Leg v6 (Autodesk Fusion 360 design; units mm, degrees)
Autodesk Fusion 360 part; units mm, degrees
sketch "RobotSatan_Outline_2" plane through (0, 0, 0) normal (0, 1, 0) x (1, 0, 0)
  spline S0 degree 3 poles (-4.0018, -2.6368) (-4.0018, -2.6368) (-1.7304, -4.4815) (0.4503, -4.3985) knots 0 0 0 0 1 1 1 1 construction
  spline S1 degree 3 poles (63.629, -4.044) (65.7695, -3.9442) (67.8342, -1.9163) (67.8342, -1.9163) knots 0 0 0 0 1 1 1 1 construction
  spline S2 degree 3 poles (61.8838, 8.3153) (62.2969, 9.5277) (62.4552, 13.6834) (61.5349, 14.1566) knots 0 0 0 0 1 1 1 1 construction
  spline S3 degree 3 poles (67.8342, -1.9163) (67.8342, -1.9163) (70.4644, 0.8212) (71.1371, 2.4758) knots 0 0 0 0 1 1 1 1 construction
  spline S4 degree 3 poles (4.7919, 41.52) (1.6976, 37.0721) (-0.1427, 30.975) (-0.3241, 24.5701) knots 0 0 0 0 1 1 1 1 construction
  spline S5 degree 3 poles (-7.7347, 1.4577) (-6.9084, -0.1335) (-4.0018, -2.6368) (-4.0018, -2.6368) knots 0 0 0 0 1 1 1 1 construction
  spline S6 degree 3 poles (25.4469, 4.8587) (26.757, 5.8451) (29.0105, 9.0389) (28.1329, 10.0991) knots 0 0 0 0 1 1 1 1 construction
  spline S7 degree 3 poles (0.9949, 13.9146) (0.1024, 13.3642) (0.6239, 9.2378) (1.1482, 8.0651) knots 0 0 0 0 1 1 1 1 construction
  line L0 (61.8838, 8.3153) -> (69.5308, 5.8795) construction
  spline S8 degree 3 poles (16.1754, 48.2878) (11.9809, 48.4024) (7.8861, 45.9679) (4.7919, 41.52) knots 0 0 0 0 1 1 1 1 construction
  spline S9 degree 3 poles (61.5349, 14.1566) (62.1985, 17.5571) (62.3292, 21.2262) (61.9169, 24.8838) knots 0 0 0 0 1 1 1 1 construction
  spline S10 degree 3 poles (-6.4002, 4.9865) (-6.4002, 4.9865) (-8.5609, 3.0488) (-7.7347, 1.4577) knots 0 0 0 0 1 1 1 1 construction
  spline S11 degree 3 poles (0.4503, -4.3985) (2.6311, -4.3154) (22.3185, -1.4309) (23.4492, 0.0355) knots 0 0 0 0 1 1 1 1 construction
  spline S12 degree 3 poles (43.7533, 47.1341) (37.1756, 46.3732) (32.0634, 39.2113) (31.0191, 29.2946) knots 0 0 0 0 1 1 1 1 construction
  line L1 (1.1482, 8.0651) -> (-6.4002, 4.9865) construction
  spline S13 degree 3 poles (71.1371, 2.4758) (71.8098, 4.1303) (69.5308, 5.8795) (69.5308, 5.8795) knots 0 0 0 0 1 1 1 1 construction
  spline S14 degree 3 poles (38.385, 3.0871) (38.9879, 1.5836) (39.975, -0.6905) (40.7508, -1.5514) knots 0 0 0 0 1 1 1 1 construction
  spline S15 degree 3 poles (40.7508, -1.5514) (41.982, -2.9178) (61.4884, -4.1438) (63.629, -4.044) knots 0 0 0 0 1 1 1 1 construction
  spline S16 degree 3 poles (-0.3241, 24.5701) (-0.4249, 20.8907) (0.0263, 17.2461) (0.9949, 13.9146) knots 0 0 0 0 1 1 1 1 construction
  spline S17 degree 3 poles (23.4492, 0.0355) (24.1617, 0.9594) (24.9655, 3.3093) (25.4469, 4.8587) knots 0 0 0 0 1 1 1 1 construction
  spline S18 degree 3 poles (31.1122, 20.9238) (31.7006, 16.2301) (33.1605, 11.7653) (35.3109, 8.0833) knots 0 0 0 0 1 1 1 1 construction
  spline S19 degree 3 poles (31.0191, 29.2946) (29.6368, 40.2178) (23.4961, 48.0751) (16.1754, 48.2878) knots 0 0 0 0 1 1 1 1 construction
  spline S20 degree 3 poles (28.1329, 10.0991) (29.6834, 13.3051) (30.7062, 17.0213) (31.1122, 20.9238) knots 0 0 0 0 1 1 1 1 construction
  spline S21 degree 3 poles (61.9169, 24.8838) (60.4852, 37.482) (53.0344, 47.225) (44.8524, 47.1981) knots 0 0 0 0 1 1 1 1 construction
  spline S22 degree 3 poles (35.3109, 8.0833) (34.543, 6.9535) (37.0192, 3.9603) (38.385, 3.0871) knots 0 0 0 0 1 1 1 1 construction
  spline S23 degree 3 poles (44.8524, 47.1981) (44.4843, 47.1969) (44.1177, 47.1755) (43.7533, 47.1341) knots 0 0 0 0 1 1 1 1 construction
  spline S24 degree 5 poles (31.0191, 29.2946) (31.0111, 29.2894) (30.9933, 29.2931) (30.9604, 29.343) (30.9015, 29.5057) (30.7982, 29.8768) (30.6618, 30.4134) (30.4903, 31.1054) (30.2828, 31.9364) (30.0394, 32.8844) (29.7611, 33.9237) (29.4494, 35.0262) (29.1066, 36.1626) (28.7352, 37.3041) (28.338, 38.4234) (27.918, 39.4965) (27.4781, 40.5035) (27.0208, 41.431) (26.5487, 42.2711) (26.0639, 43.0212) (25.5684, 43.6827) (25.0637, 44.2606) (24.5515, 44.7626) (24.0328, 45.1982) (23.5086, 45.5782) (22.9796, 45.9134) (22.4464, 46.2145) (21.909, 46.4908) (21.3676, 46.7496) (20.8219, 46.9954) (20.2714, 47.2296) (19.7155, 47.4512) (19.1536, 47.6575) (18.585, 47.8443) (18.0094, 48.0066) (17.4263, 48.1391) (16.8357, 48.2366) (16.2379, 48.2949) (15.6336, 48.3107) (15.0238, 48.2827) (14.4104, 48.2111) (13.795, 48.0973) (13.1799, 47.9437) (12.5675, 47.7532) (11.96, 47.5293) (11.3598, 47.2753) (10.7691, 46.9943) (10.1899, 46.6888) (9.624, 46.3606) (9.0726, 46.0102) (8.5367, 45.6368) (8.017, 45.2393) (7.5137, 44.8154) (7.0269, 44.363) (6.5565, 43.8795) (6.102, 43.3625) (5.6629, 42.8101) (5.2387, 42.2208) (4.8287, 41.5939) (4.4321, 40.9297) (4.0482, 40.23) (3.6763, 39.4975) (3.3159, 38.7358) (2.9663, 37.9493) (2.6273, 37.1425) (2.2986, 36.3207) (1.9802, 35.4888) (1.6724, 34.6516) (1.3757, 33.8137) (1.0908, 32.9788) (0.8191, 32.1501) (0.562, 31.3295) (0.3215, 30.5177) (0.1, 29.7142) (-0.0996, 28.9165) (-0.2743, 28.1212) (-0.4207, 27.3241) (-0.536, 26.5206) (-0.6172, 25.7065) (-0.6623, 24.8778) (-0.6696, 24.0319) (-0.6387, 23.1674) (-0.5701, 22.2848) (-0.4654, 21.387) (-0.3281, 20.4794) (-0.1632, 19.571) (0.0225, 18.6739) (0.2201, 17.8048) (0.4185, 16.9835) (0.6063, 16.231) (0.7719, 15.5667) (0.9049, 15.0065) (0.9968, 14.5606) (1.042, 14.2311) (1.0388, 14.0095) (0.9901, 13.8752) (0.9047, 13.7922) (0.7973, 13.7097) (0.6851, 13.5785) (0.5842, 13.3649) (0.5088, 13.0503) (0.4701, 12.6295) (0.4753, 12.1101) (0.5262, 11.5114) (0.6185, 10.8629) (0.7407, 10.204) (0.876, 9.578) (1.0052, 9.0265) (1.1093, 8.5838) (1.1717, 8.2713) (1.1807, 8.0912) (1.1322, 8.0228) (1.0327, 8.0115) (0.8972, 7.9857) (0.7382, 7.921) (0.5625, 7.8283) (0.369, 7.728) (0.1458, 7.6264) (-0.1255, 7.5178) (-0.4648, 7.3903) (-0.8886, 7.2301) (-1.4057, 7.0265) (-2.0115, 6.7767) (-2.6848, 6.4899) (-3.3936, 6.1826) (-4.0992, 5.876) (-4.7615, 5.5924) (-5.3435, 5.352) (-5.8163, 5.1692) (-6.1636, 5.05) (-6.3871, 4.9878) (-6.5098, 4.9612) (-6.5847, 4.9281) (-6.6707, 4.8433) (-6.7961, 4.6861) (-6.9627, 4.4573) (-7.1567, 4.1701) (-7.3567, 3.8446) (-7.5443, 3.4995) (-7.7054, 3.15) (-7.8298, 2.8085) (-7.9105, 2.4837) (-7.9435, 2.1803) (-7.9276, 1.899) (-7.8635, 1.6359) (-7.754, 1.3841) (-7.6034, 1.1356) (-7.417, 0.8829) (-7.2008, 0.6209) (-6.9611, 0.3474) (-6.7041, 0.0626) (-6.4358, -0.2313) (-6.1612, -0.5311) (-5.8841, -0.8324) (-5.6068, -1.1306) (-5.33, -1.4212) (-5.0532, -1.7) (-4.776, -1.9634) (-4.4979, -2.2088) (-4.2193, -2.4347) (-3.9422, -2.6411) (-3.6705, -2.8298) (-3.4086, -3.0036) (-3.1594, -3.1658) (-2.9235, -3.3194) (-2.6971, -3.4672) (-2.4707, -3.6101) (-2.2323, -3.7483) (-1.9713, -3.8807) (-1.6808, -4.0054) (-1.3626, -4.1197) (-1.0273, -4.2204) (-0.6894, -4.3043) (-0.3635, -4.3684) (-0.06, -4.4107) (0.2192, -4.4301) (0.4846, -4.4277) (0.7549, -4.4053) (1.0522, -4.3659) (1.3972, -4.3126) (1.8047, -4.2485) (2.2802, -4.1762) (2.8216, -4.098) (3.4209, -4.0156) (4.0658, -3.9307) (4.7411, -3.8444) (5.4302, -3.7577) (6.1166, -3.6711) (6.7858, -3.5852) (7.4264, -3.5002) (8.0317, -3.4161) (8.6006, -3.3329) (9.1356, -3.2504) (9.6424, -3.1682) (10.1289, -3.0859) (10.6041, -3.0031) (11.0773, -2.9193) (11.557, -2.8339) (12.0504, -2.7463) (12.5617, -2.6561) (13.0932, -2.5628) (13.645, -2.4658) (14.2157, -2.365) (14.8026, -2.2599) (15.4022, -2.1504) (16.01, -2.0365) (16.6217, -1.9183) (17.2328, -1.7961) (17.8392, -1.6704) (18.4372, -1.5419) (19.0234, -1.4113) (19.5943, -1.2794) (20.1462, -1.1472) (20.6751, -1.0154) (21.1762, -0.8847) (21.6444, -0.7558) (22.0732, -0.629) (22.4551, -0.5047) (22.7823, -0.3827) (23.0491, -0.2627) (23.2538, -0.144) (23.4009, -0.0255) (23.5034, 0.0941) (23.5821, 0.2169) (23.6573, 0.3472) (23.7421, 0.4931) (23.8421, 0.6649) (23.9589, 0.8736) (24.0916, 1.1286) (24.238, 1.4367) (24.3945, 1.8003) (24.5567, 2.2164) (24.7193, 2.6747) (24.8766, 3.1566) (25.0229, 3.6331) (25.153, 4.0687) (25.2636, 4.4304) (25.3547, 4.6943) (25.431, 4.8544) (25.5023, 4.9287) (25.5865, 4.9705) (25.702, 5.0425) (25.8576, 5.1765) (26.0542, 5.3795) (26.2863, 5.643) (26.5442, 5.9509) (26.8158, 6.2885) (27.0881, 6.6445) (27.3482, 7.0094) (27.5846, 7.3755) (27.7883, 7.7361) (27.9542, 8.0852) (28.082, 8.4167) (28.1777, 8.7241) (28.2497, 9.0014) (28.3043, 9.2445) (28.3428, 9.452) (28.3543, 9.6267) (28.3198, 9.7759) (28.2352, 9.9073) (28.1424, 10.0247) (28.1125, 10.1292) (28.1686, 10.2278) (28.2589, 10.336) (28.3384, 10.4699) (28.4062, 10.6416) (28.4793, 10.8573) (28.5744, 11.1149) (28.6922, 11.4037) (28.8257, 11.7082) (28.9627, 12.0126) (29.0913, 12.3043) (29.2043, 12.5783) (29.3022, 12.8394) (29.3899, 13.0974) (29.4739, 13.3628) (29.5603, 13.6434) (29.6516, 13.939) (29.7464, 14.2424) (29.8414, 14.544) (29.9328, 14.8349) (30.0175, 15.1108) (30.0953, 15.3768) (30.1682, 15.6452) (30.2391, 15.9303) (30.3112, 16.2431) (30.386, 16.5867) (30.4628, 16.9503) (30.5386, 17.3134) (30.61, 17.654) (30.6737, 17.9546) (30.7279, 18.209) (30.7735, 18.4304) (30.8143, 18.6527) (30.8548, 18.9132) (30.8989, 19.2396) (30.948, 19.6357) (30.9989, 20.0659) (31.046, 20.471) (31.084, 20.7851) (31.1099, 20.9528) (31.125, 20.9445) (31.1381, 20.7771) (31.1614, 20.4992) (31.2015, 20.1593) (31.257, 19.7928) (31.3225, 19.425) (31.3901, 19.0714) (31.4534, 18.7382) (31.5088, 18.4237) (31.5597, 18.1183) (31.6142, 17.8079) (31.6818, 17.4778) (31.7711, 17.1163) (31.8868, 16.7185) (32.0268, 16.2903) (32.18, 15.8506) (32.3309, 15.4247) (32.4634, 15.0385) (32.5644, 14.7123) (32.6277, 14.455) (32.6576, 14.2585) (32.6737, 14.09) (32.7019, 13.9064) (32.7645, 13.671) (32.8676, 13.3723) (33.0016, 13.0247) (33.1492, 12.6556) (33.2908, 12.297) (33.4115, 11.9747) (33.5072, 11.6991) (33.5911, 11.4551) (33.6858, 11.2126) (33.8153, 10.9375) (33.9976, 10.6027) (34.2358, 10.1988) (34.5114, 9.7444) (34.7924, 9.2758) (35.0416, 8.8367) (35.2248, 8.4679) (35.3196, 8.1968) (35.3223, 8.0283) (35.2592, 7.9314) (35.186, 7.8396) (35.1473, 7.7015) (35.1511, 7.5126) (35.1875, 7.2909) (35.2458, 7.0538) (35.327, 6.8025) (35.4373, 6.5302) (35.5855, 6.2274) (35.779, 5.8874) (36.0193, 5.5123) (36.3012, 5.1148) (36.6145, 4.7134) (36.9452, 4.3294) (37.2769, 3.9837) (37.592, 3.6931) (37.8734, 3.4674) (38.1053, 3.3053) (38.2753, 3.193) (38.3802, 3.1082) (38.4305, 3.0249) (38.4579, 2.9172) (38.5006, 2.7655) (38.5761, 2.5645) (38.6835, 2.3206) (38.8123, 2.0468) (38.9486, 1.7575) (39.0838, 1.4639) (39.2143, 1.1727) (39.34, 0.8879) (39.4637, 0.6104) (39.5892, 0.3391) (39.7204, 0.0711) (39.8606, -0.1965) (40.0108, -0.4652) (40.1698, -0.7325) (40.3324, -0.9907) (40.4887, -1.2241) (40.6273, -1.4141) (40.741, -1.5488) (40.8312, -1.629) (40.9141, -1.679) (41.0117, -1.7285) (41.1388, -1.7875) (41.3038, -1.8535) (41.5087, -1.9227) (41.7511, -1.9933) (42.0259, -2.0637) (42.3276, -2.1336) (42.6519, -2.2027) (42.9967, -2.2709) (43.3612, -2.3383) (43.7457, -2.4051) (44.1511, -2.4716) (44.5782, -2.5378) (45.0279, -2.604) (45.5003, -2.6699) (45.9952, -2.7356) (46.5116, -2.8008) (47.0479, -2.8653) (47.602, -2.9287) (48.1709, -2.9909) (48.7506, -3.0514) (49.3364, -3.1101) (49.9228, -3.1667) (50.5038, -3.2211) (51.0735, -3.2731) (51.6264, -3.3227) (52.1582, -3.3698) (52.6659, -3.4144) (53.1483, -3.4565) (53.6066, -3.4962) (54.0446, -3.5336) (54.4691, -3.5688) (54.8881, -3.6021) (55.3097, -3.6335) (55.7415, -3.6634) (56.1886, -3.6921) (56.6534, -3.7199) (57.1335, -3.7472) (57.6219, -3.7745) (58.109, -3.8022) (58.5841, -3.8304) (59.0372, -3.8593) (59.4608, -3.8885) (59.8514, -3.9176) (60.2118, -3.9454) (60.5522, -3.9705) (60.887, -3.991) (61.2307, -4.0058) (61.594, -4.0141) (61.9799, -4.0166) (62.3794, -4.0153) (62.7692, -4.0144) (63.1214, -4.0177) (63.4113, -4.0275) (63.6264, -4.0427) (63.7743, -4.0574) (63.8925, -4.0584) (64.0263, -4.0338) (64.1962, -3.9855) (64.394, -3.927) (64.6018, -3.8725) (64.8064, -3.8247) (65.0063, -3.7731) (65.205, -3.7041) (65.4083, -3.6083) (65.6205, -3.4881) (65.8441, -3.3521) (66.0797, -3.2104) (66.3259, -3.0689) (66.5791, -2.9242) (66.834, -2.7677) (67.0841, -2.5905) (67.3228, -2.3881) (67.5437, -2.1655) (67.7412, -1.9413) (67.912, -1.7384) (68.0567, -1.5756) (68.1802, -1.46) (68.2946, -1.3756) (68.4141, -1.2927) (68.5485, -1.1848) (68.6977, -1.0404) (68.8564, -0.8598) (69.0166, -0.6528) (69.1722, -0.4364) (69.3198, -0.2295) (69.4587, -0.0462) (69.5911, 0.1099) (69.723, 0.2541) (69.8617, 0.413) (70.0127, 0.6105) (70.1758, 0.8543) (70.3431, 1.125) (70.5029, 1.3906) (70.6441, 1.619) (70.7595, 1.7903) (70.8514, 1.9138) (70.93, 2.0231) (71.0047, 2.1513) (71.0769, 2.3071) (71.142, 2.4806) (71.1947, 2.6563) (71.2328, 2.8234) (71.256, 2.978) (71.2649, 3.1263) (71.2596, 3.2836) (71.2402, 3.4608) (71.2062, 3.6458) (71.1575, 3.8109) (71.0967, 3.9366) (71.0318, 4.0377) (70.9712, 4.1506) (70.9096, 4.2933) (70.8309, 4.4574) (70.7255, 4.6233) (70.609, 4.771) (70.5069, 4.8902) (70.429, 4.987) (70.3414, 5.0957) (70.1989, 5.253) (69.9874, 5.4655) (69.7602, 5.6833) (69.5848, 5.8436) (69.5049, 5.9042) (69.4785, 5.8941) (69.377, 5.9175) (69.2074, 5.9796) (69.0289, 6.0454) (68.8687, 6.0968) (68.7112, 6.1417) (68.5308, 6.1943) (68.3148, 6.2617) (68.0659, 6.3427) (67.7933, 6.4325) (67.5087, 6.5252) (67.2182, 6.6179) (66.9232, 6.7108) (66.6226, 6.8053) (66.3152, 6.903) (66.0018, 7.0044) (65.6877, 7.107) (65.382, 7.2064) (65.0949, 7.2978) (64.8344, 7.3776) (64.6044, 7.4453) (64.401, 7.5052) (64.2136, 7.5653) (64.0269, 7.6331) (63.8224, 7.7128) (63.5816, 7.8026) (63.2922, 7.8974) (62.9553, 7.9908) (62.5906, 8.0774) (62.246, 8.1547) (61.9895, 8.2246) (61.8649, 8.2894) (61.8793, 8.3527) (61.9283, 8.4107) (61.9329, 8.4774) (61.9545, 8.5927) (61.995, 8.7507) (62.0358, 8.9242) (62.0638, 9.0923) (62.0829, 9.2506) (62.1005, 9.4028) (62.1198, 9.5578) (62.1391, 9.7238) (62.156, 9.9023) (62.1699, 10.0834) (62.1812, 10.2552) (62.1905, 10.4139) (62.1981, 10.5706) (62.2043, 10.7396) (62.209, 10.9281) (62.2118, 11.1312) (62.2124, 11.3395) (62.2103, 11.543) (62.205, 11.7356) (62.1964, 11.9151) (62.185, 12.0848) (62.1722, 12.2534) (62.1588, 12.4287) (62.1431, 12.6089) (62.1211, 12.7795) (62.0909, 12.9272) (62.0592, 13.0553) (62.0392, 13.1869) (62.0281, 13.342) (61.991, 13.5221) (61.894, 13.7146) (61.7371, 13.8994) (61.586, 14.0537) (61.5113, 14.1632) (61.5386, 14.2322) (61.5778, 14.2953) (61.5869, 14.3962) (61.6011, 14.5685) (61.6368, 14.8098) (61.6892, 15.0879) (61.7447, 15.3626) (61.7887, 15.6) (61.8174, 15.7946) (61.8365, 15.9635) (61.8543, 16.1294) (61.8757, 16.3032) (61.8996, 16.4804) (61.9233, 16.6553) (61.9453, 16.8339) (61.9665, 17.035) (61.9881, 17.2795) (62.0115, 17.5833) (62.0368, 17.9499) (62.0633, 18.3744) (62.0899, 18.8455) (62.115, 19.3479) (62.1367, 19.8655) (62.1532, 20.3834) (62.1631, 20.8908) (62.1649, 21.3832) (62.158, 21.8608) (62.1419, 22.3275) (62.1162, 22.7894) (62.0812, 23.2534) (62.0372, 23.726) (61.9849, 24.212) (61.9251, 24.7129) (61.859, 25.2265) (61.7875, 25.7479) (61.712, 26.2706) (61.6333, 26.7872) (61.5524, 27.2906) (61.4696, 27.7751) (61.3852, 28.2367) (61.2988, 28.675) (61.2092, 29.0932) (61.115, 29.4977) (61.0147, 29.8963) (60.9062, 30.298) (60.7877, 30.7111) (60.6575, 31.1431) (60.5142, 31.5991) (60.3566, 32.081) (60.1842, 32.5883) (59.9967, 33.1182) (59.794, 33.6667) (59.5765, 34.2283) (59.3449, 34.7973) (59.0998, 35.3676) (58.8426, 35.9335) (58.5743, 36.4903) (58.2966, 37.0343) (58.011, 37.5633) (57.719, 38.076) (57.4219, 38.5719) (57.1209, 39.0512) (56.8166, 39.515) (56.5094, 39.9643) (56.1987, 40.4008) (55.8836, 40.8262) (55.5622, 41.2421) (55.2317, 41.6502) (54.8893, 42.0517) (54.5317, 42.4476) (54.156, 42.8387) (53.7597, 43.2251) (53.3407, 43.6066) (52.8982, 43.9821) (52.4322, 44.3499) (51.9447, 44.7075) (51.4384, 45.0519) (50.9173, 45.3796) (50.3859, 45.687) (49.8489, 45.9705) (49.3114, 46.227) (48.7781, 46.4538) (48.2529, 46.6492) (47.7394, 46.8123) (47.2396, 46.9436) (46.7547, 47.0446) (46.2845, 47.1182) (45.828, 47.1671) (45.3838, 47.1945) (44.9496, 47.2033) (44.5229, 47.1955) (44.1009, 47.1722) (43.6811, 47.133) (43.2608, 47.0762) (42.8379, 46.9997) (42.4105, 46.9009) (41.9777, 46.7777) (41.5394, 46.6284) (41.0964, 46.4526) (40.651, 46.2514) (40.2062, 46.0273) (39.7658, 45.7836) (39.3338, 45.5239) (38.914, 45.2519) (38.5097, 44.9708) (38.1234, 44.683) (37.7562, 44.3893) (37.4076, 44.0891) (37.0759, 43.78) (36.7584, 43.4591) (36.4519, 43.123) (36.1533, 42.7686) (35.8596, 42.3938) (35.5689, 41.9975) (35.2804, 41.5808) (34.9945, 41.1466) (34.7128, 40.6994) (34.4376, 40.2445) (34.1715, 39.7873) (33.9172, 39.3332) (33.6772, 38.8863) (33.4533, 38.4496) (33.2466, 38.024) (33.0569, 37.6077) (32.883, 37.1974) (32.7233, 36.7885) (32.5756, 36.3763) (32.4375, 35.9568) (32.3067, 35.527) (32.1813, 35.086) (32.0601, 34.6359) (31.9421, 34.1808) (31.8273, 33.7266) (31.716, 33.2791) (31.6089, 32.8438) (31.5074, 32.4249) (31.4131, 32.024) (31.3279, 31.6394) (31.2541, 31.2664) (31.1934, 30.9005) (31.1467, 30.5399) (31.1132, 30.1881) (31.0904, 29.8569) (31.0731, 29.5691) (31.0576, 29.4003) (31.0412, 29.3241) (31.0271, 29.2998) (31.0191, 29.2946) knots 0 0 0 0 0 0 0.00138889 0.00277778 0.00416667 0.00555556 0.00694444 0.00833333 0.00972222 0.01111111 0.0125 0.01388889 0.01527778 0.01666667 0.01805556 0.01944444 0.02083333 0.02222222 0.02361111 0.025 0.02638889 0.02777778 0.02916667 0.03055556 0.03194444 0.03333333 0.03472222 0.03611111 0.0375 0.03888889 0.04027778 0.04166667 0.04305556 0.04444444 0.04583333 0.04722222 0.04861111 0.05 0.05138889 0.05277778 0.05416667 0.05555556 0.05694444 0.05833333 0.05972222 0.06111111 0.0625 0.06388889 0.06527778 0.06666667 0.06805556 0.06944444 0.07083333 0.07222222 0.07361111 0.075 0.07638889 0.07777778 0.07916667 0.08055556 0.08194444 0.08333333 0.08472222 0.08611111 0.0875 0.08888889 0.09027778 0.09166667 0.09305556 0.09444444 0.09583333 0.09722222 0.09861111 0.1 0.10138889 0.10277778 0.10416667 0.10555556 0.10694444 0.10833333 0.10972222 0.11111111 0.1125 0.11388889 0.11527778 0.11666667 0.11805556 0.11944444 0.12083333 0.12222222 0.12361111 0.125 0.12638889 0.12777778 0.12916667 0.13055556 0.13194444 0.13333333 0.13472222 0.13611111 0.1375 0.13888889 0.14027778 0.14166667 0.14305556 0.14444444 0.14583333 0.14722222 0.14861111 0.15 0.15138889 0.15277778 0.15416667 0.15555556 0.15694444 0.15833333 0.15972222 0.16111111 0.1625 0.16388889 0.16527778 0.16666667 0.16805556 0.16944444 0.17083333 0.17222222 0.17361111 0.175 0.17638889 0.17777778 0.17916667 0.18055556 0.18194444 0.18333333 0.18472222 0.18611111 0.1875 0.18888889 0.19027778 0.19166667 0.19305556 0.19444444 0.19583333 0.19722222 0.19861111 0.2 0.20138889 0.20277778 0.20416667 0.20555556 0.20694444 0.20833333 0.20972222 0.21111111 0.2125 0.21388889 0.21527778 0.21666667 0.21805556 0.21944444 0.22083333 0.22222222 0.22361111 0.225 0.22638889 0.22777778 0.22916667 0.23055556 0.23194444 0.23333333 0.23472222 0.23611111 0.2375 0.23888889 0.24027778 0.24166667 0.24305556 0.24444444 0.24583333 0.24722222 0.24861111 0.25 0.25138889 0.25277778 0.25416667 0.25555556 0.25694444 0.25833333 0.25972222 0.26111111 0.2625 0.26388889 0.26527778 0.26666667 0.26805556 0.26944444 0.27083333 0.27222222 0.27361111 0.275 0.27638889 0.27777778 0.27916667 0.28055556 0.28194444 0.28333333 0.28472222 0.28611111 0.2875 0.28888889 0.29027778 0.29166667 0.29305556 0.29444444 0.29583333 0.29722222 0.29861111 0.3 0.30138889 0.30277778 0.30416667 0.30555556 0.30694444 0.30833333 0.30972222 0.31111111 0.3125 0.31388889 0.31527778 0.31666667 0.31805556 0.31944444 0.32083333 0.32222222 0.32361111 0.325 0.32638889 0.32777778 0.32916667 0.33055556 0.33194444 0.33333333 0.33472222 0.33611111 0.3375 0.33888889 0.34027778 0.34166667 0.34305556 0.34444444 0.34583333 0.34722222 0.34861111 0.35 0.35138889 0.35277778 0.35416667 0.35555556 0.35694444 0.35833333 0.35972222 0.36111111 0.3625 0.36388889 0.36527778 0.36666667 0.36805556 0.36944444 0.37083333 0.37222222 0.37361111 0.375 0.37638889 0.37777778 0.37916667 0.38055556 0.38194444 0.38333333 0.38472222 0.38611111 0.3875 0.38888889 0.39027778 0.39166667 0.39305556 0.39444444 0.39583333 0.39722222 0.39861111 0.4 0.40138889 0.40277778 0.40416667 0.40555556 0.40694444 0.40833333 0.40972222 0.41111111 0.4125 0.41388889 0.41527778 0.41666667 0.41805556 0.41944444 0.42083333 0.42222222 0.42361111 0.425 0.42638889 0.42777778 0.42916667 0.43055556 0.43194444 0.43333333 0.43472222 0.43611111 0.4375 0.43888889 0.44027778 0.44166667 0.44305556 0.44444444 0.44583333 0.44722222 0.44861111 0.45 0.45138889 0.45277778 0.45416667 0.45555556 0.45694444 0.45833333 0.45972222 0.46111111 0.4625 0.46388889 0.46527778 0.46666667 0.46805556 0.46944444 0.47083333 0.47222222 0.47361111 0.475 0.47638889 0.47777778 0.47916667 0.48055556 0.48194444 0.48333333 0.48472222 0.48611111 0.4875 0.48888889 0.49027778 0.49166667 0.49305556 0.49444444 0.49583333 0.49722222 0.49861111 0.5 0.50138889 0.50277778 0.50416667 0.50555556 0.50694444 0.50833333 0.50972222 0.51111111 0.5125 0.51388889 0.51527778 0.51666667 0.51805556 0.51944444 0.52083333 0.52222222 0.52361111 0.525 0.52638889 0.52777778 0.52916667 0.53055556 0.53194444 0.53333333 0.53472222 0.53611111 0.5375 0.53888889 0.54027778 0.54166667 0.54305556 0.54444444 0.54583333 0.54722222 0.54861111 0.55 0.55138889 0.55277778 0.55416667 0.55555556 0.55694444 0.55833333 0.55972222 0.56111111 0.5625 0.56388889 0.56527778 0.56666667 0.56805556 0.56944444 0.57083333 0.57222222 0.57361111 0.575 0.57638889 0.57777778 0.57916667 0.58055556 0.58194444 0.58333333 0.58472222 0.58611111 0.5875 0.58888889 0.59027778 0.59166667 0.59305556 0.59444444 0.59583333 0.59722222 0.59861111 0.6 0.60138889 0.60277778 0.60416667 0.60555556 0.60694444 0.60833333 0.60972222 0.61111111 0.6125 0.61388889 0.61527778 0.61666667 0.61805556 0.61944444 0.62083333 0.62222222 0.62361111 0.625 0.62638889 0.62777778 0.62916667 0.63055556 0.63194444 0.63333333 0.63472222 0.63611111 0.6375 0.63888889 0.64027778 0.64166667 0.64305556 0.64444444 0.64583333 0.64722222 0.64861111 0.65 0.65138889 0.65277778 0.65416667 0.65555556 0.65694444 0.65833333 0.65972222 0.66111111 0.6625 0.66388889 0.66527778 0.66666667 0.66805556 0.66944444 0.67083333 0.67222222 0.67361111 0.675 0.67638889 0.67777778 0.67916667 0.68055556 0.68194444 0.68333333 0.68472222 0.68611111 0.6875 0.68888889 0.69027778 0.69166667 0.69305556 0.69444444 0.69583333 0.69722222 0.69861111 0.7 0.70138889 0.70277778 0.70416667 0.70555556 0.70694444 0.70833333 0.70972222 0.71111111 0.7125 0.71388889 0.71527778 0.71666667 0.71805556 0.71944444 0.72083333 0.72222222 0.72361111 0.725 0.72638889 0.72777778 0.72916667 0.73055556 0.73194444 0.73333333 0.73472222 0.73611111 0.7375 0.73888889 0.74027778 0.74166667 0.74305556 0.74444444 0.74583333 0.74722222 0.74861111 0.75 0.75138889 0.75277778 0.75416667 0.75555556 0.75694444 0.75833333 0.75972222 0.76111111 0.7625 0.76388889 0.76527778 0.76666667 0.76805556 0.76944444 0.77083333 0.77222222 0.77361111 0.775 0.77638889 0.77777778 0.77916667 0.78055556 0.78194444 0.78333333 0.78472222 0.78611111 0.7875 0.78888889 0.79027778 0.79166667 0.79305556 0.79444444 0.79583333 0.79722222 0.79861111 0.8 0.80138889 0.80277778 0.80416667 0.80555556 0.80694444 0.80833333 0.80972222 0.81111111 0.8125 0.81388889 0.81527778 0.81666667 0.81805556 0.81944444 0.82083333 0.82222222 0.82361111 0.825 0.82638889 0.82777778 0.82916667 0.83055556 0.83194444 0.83333333 0.83472222 0.83611111 0.8375 0.83888889 0.84027778 0.84166667 0.84305556 0.84444444 0.84583333 0.84722222 0.84861111 0.85 0.85138889 0.85277778 0.85416667 0.85555556 0.85694444 0.85833333 0.85972222 0.86111111 0.8625 0.86388889 0.86527778 0.86666667 0.86805556 0.86944444 0.87083333 0.87222222 0.87361111 0.875 0.87638889 0.87777778 0.87916667 0.88055556 0.88194444 0.88333333 0.88472222 0.88611111 0.8875 0.88888889 0.89027778 0.89166667 0.89305556 0.89444444 0.89583333 0.89722222 0.89861111 0.9 0.90138889 0.90277778 0.90416667 0.90555556 0.90694444 0.90833333 0.90972222 0.91111111 0.9125 0.91388889 0.91527778 0.91666667 0.91805556 0.91944444 0.92083333 0.92222222 0.92361111 0.925 0.92638889 0.92777778 0.92916667 0.93055556 0.93194444 0.93333333 0.93472222 0.93611111 0.9375 0.93888889 0.94027778 0.94166667 0.94305556 0.94444444 0.94583333 0.94722222 0.94861111 0.95 0.95138889 0.95277778 0.95416667 0.95555556 0.95694444 0.95833333 0.95972222 0.96111111 0.9625 0.96388889 0.96527778 0.96666667 0.96805556 0.96944444 0.97083333 0.97222222 0.97361111 0.975 0.97638889 0.97777778 0.97916667 0.98055556 0.98194444 0.98333333 0.98472222 0.98611111 0.9875 0.98888889 0.99027778 0.99166667 0.99305556 0.99444444 0.99583333 0.99722222 0.99861111 1 1 1 1 1 1
  line L2 (31.1533, 48.967) -> (31.1533, -17) construction
  line L3 (-18.8467, 30.6015) -> (81.1533, 30.6015) construction
  circle A0 centre (6.1533, 30.6015) radius 1.5
  circle A1 centre (56.1533, 30.6015) radius 1.5
  point P0 (0.0049, 0)
  point P1 (-320.2084, 0)
  point P2 (21080909.6473, 0)
  point P3 (0.0049, 0)
  point P4 (0, 0)
  point P5 (0, 0)
  dimension "d3" = 25
  dimension "d4" = 25
  dimension "d5" = 3
  dimension "d6" = 3
  dimension "d7" = 100
  dimension "d8" = 50
  dimension "d9" = 35
  constraint coincident S18
  constraint coincident S22
  constraint coincident S22 P5
  constraint coincident S14 P5
  constraint coincident S14
  constraint coincident S15
  constraint coincident S15 P5
  constraint coincident S15 P2
  constraint coincident L0 P5
  constraint coincident L0 P3
  constraint coincident L0
  constraint coincident S2
  constraint coincident S2 P5
  constraint coincident S9 P5
  constraint coincident S9
  constraint coincident S21
  constraint coincident S21 P5
  constraint coincident S23 P5
  constraint coincident S12 P5
  constraint coincident S12
  constraint vertical L2
  constraint horizontal L3
  constraint coincident L3 P5
  measures "d5" diameter of A0
  measures "d6" diameter of A1
extrude "Extrude1" add sketch "RobotSatan_Outline_2" along normal blind 3 contours S24 | A0 | A1 makes body 1
extrude "Extrude2" add sketch "RobotSatan_Outline_2" against normal blind 3 separate body contours A0 | A1 makes body 2 at (7.6515, -2, -30.5268) makes body 3 at (55.469, -2, -29.2667)
